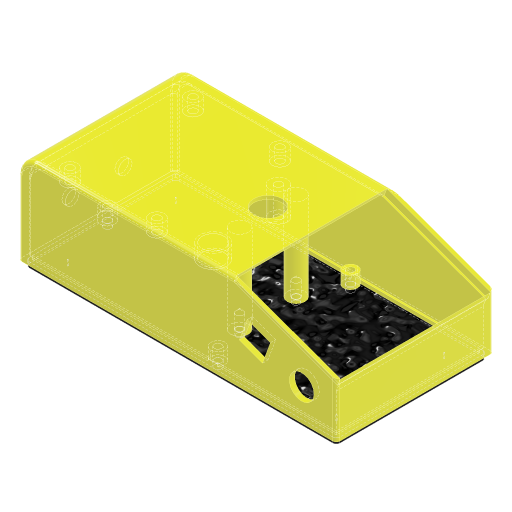
# Autodesk Inventor part: gabinete6
Saved by Autodesk Inventor 2023 (Build 270158000, 158)
## iProperties
Created: 2023-09-18
Part Number: gabinete6
Material: Generic
Document SubType Name: Modeling
Designer: Claudimir
Density: 1 g/cm^3
Appearance: Default
Author: Claudimir
Autodesk Inventor part; units mm, degrees
ref_plane "YZ Plane" through (0, 0, 0) normal (1, 0, 0) x (0, 1, 0)
ref_plane "XZ Plane" through (0, 0, 0) normal (0, 1, 0) x (-1, 0, 0)
sketch "Sketch1" plane through (0, 0, 0) normal (0, 0, 1) x (1, 0, 0)
  line L0 (0, 0) -> (9.2345, 25.3717) construction
  line L1 (9.2345, 25.3717) -> (-49.0264, 46.5769)
  line L2 (-49.0264, 46.5769) -> (-58.2609, 21.2052) construction
  line L3 (-58.2609, 21.2052) -> (0, 0) construction
  line L4 (-49.0264, 46.5769) -> (-53.6437, 33.8911) construction
  line L5 (-53.6437, 33.8911) -> (-40.9578, 29.2738) construction
  line L6 (-40.9578, 29.2738) -> (-36.3405, 41.9597) construction
  line L7 (-36.3405, 41.9597) -> (-49.0264, 46.5769) construction
  line L8 (-40.9578, 29.2738) -> (-45.0621, 17.9975) construction
  line L9 (-45.0621, 17.9975) -> (-32.8461, 13.5513) construction
  line L10 (-32.8461, 13.5513) -> (-28.7418, 24.8276) construction
  line L11 (-28.7418, 24.8276) -> (-40.9578, 29.2738) construction
  line L12 (9.2345, 25.3717) -> (4.4463, 12.216) construction
  line L13 (4.4463, 12.216) -> (-4.011, 15.2942) construction
  line L14 (-4.011, 15.2942) -> (0.7773, 28.4499) construction
  line L15 (0.7773, 28.4499) -> (9.2345, 25.3717) construction
  line L16 (-4.011, 15.2942) -> (-7.4312, 5.8973) construction
  line L17 (-7.4312, 5.8973) -> (-16.8281, 9.3175) construction
  line L18 (-16.8281, 9.3175) -> (-13.4079, 18.7144) construction
  line L19 (-13.4079, 18.7144) -> (-4.011, 15.2942) construction
  line L20 (-170.7655, -8.4231) -> (9.2345, -8.4231)
  line L21 (9.2345, -8.4231) -> (9.2345, 25.3717)
  line L22 (-49.0264, 46.5769) -> (-170.7655, 46.5769)
  line L23 (-45.7029, 17.6987) -> (-41.2567, 29.9147)
  line L24 (-41.2567, 29.9147) -> (-28.101, 25.1264)
  line L25 (-28.101, 25.1264) -> (-32.5472, 12.9104)
  line L26 (-32.5472, 12.9104) -> (-45.7029, 17.6987)
  line L27 (-13.4079, 18.7144) -> (-7.4312, 5.8973) construction
  line L28 (-4.011, 15.2942) -> (-16.8281, 9.3175) construction
  circle A0 centre (-10.4195, 12.3058) radius 7
  line L29 (-170.7655, 46.5769) -> (-170.7655, -8.4231)
  line L30 (-168.7655, 44.5769) -> (-49.7543, 44.5769)
  line L31 (6.2345, 17.1293) -> (6.2345, -8.4231)
  line L32 (-168.7655, -8.4231) -> (-168.7655, 44.5769)
  line L33 (-49.7543, 44.5769) -> (-49.0264, 46.5769)
  line L34 (6.2345, 17.1293) -> (9.2345, 25.3717)
  point P0 (6.2345, -8.4231)
  dimension "d0" = 27
  dimension "d1" = 62
  dimension "d4" = 12
  dimension "d5" = 13
  dimension "d6" = 14
  dimension "d7" = 9
  dimension "d8" = 10
  dimension "d9" = 10
  dimension "d13" = 180
  dimension "d17" = 0.5
  dimension "d18" = 14
  dimension "d19" = 55
  dimension "d22" = 2
  constraints: 70 end point, 13 parallel, 6 perpendicular, 3 point on line, 1 centre point, 1 collinear, 1 horizontal, 1 midpoint, 1 vertical, 5 other
  measures "d0" distance of L2.end L1.end
  measures "d1" distance of L1.end L0.end
  measures "d4" distance of L10.end L9.end
  measures "d5" distance of L9.end L8.end
  measures "d6" distance of L13.end L14.end
  measures "d7" distance of L12.end L13.end
  measures "d8" distance of L17.end L18.end
  measures "d9" distance of L16.end L17.end
  measures "d13" distance of L20.end L20.start
  measures "d17" distance between parallel lines of L8 L23
  measures "d18" diameter of A0
  measures "d19" distance of L22.end L20.start
  measures "d22" distance between parallel lines of L22 L30
extrude "corpo 1" add sketch "Sketch1" against normal blind 89 contours L34 L31 L20 L32 L30 L33 L1 | L21 L20 L31 L34 | L33 L30 L32 L20 L29 L22 | L23 L24 L25 L26 | A0
extrude "corpo 2" cut sketch "Sketch1" against normal blind 86 contours L34 L31 L20 L32 L30 L33 L1 | L23 L24 L25 L26 | A0
extrude "corpo 3" add sketch "Sketch1" against normal blind 3
sketch "Sketch2" plane through (-170.7655, 46.5769, -89) normal (0, 1, 0) x (1, 0, 0)
  line L0 (121.7391, 0) -> (180, 0) construction
  line L1 (121.7391, 0) -> (96.7391, 0) construction
  line L2 (96.7391, 0) -> (96.7391, -44.5) construction
  line L3 (96.7391, -44.5) -> (121.7391, -44.5) construction
  line L4 (121.7391, -44.5) -> (121.7391, 0) construction
  circle A0 centre (96.7391, -44.5) radius 8
  point P0 (170.7655, -89)
  dimension "d27" = 25
  dimension "d28" = 44.5
  dimension "d29" = 16
  constraints: 8 end point, 2 parallel, 1 centre point, 1 coincident, 1 horizontal, 1 perpendicular
  measures "d27" distance of L3.end L2.end
  measures "d28" distance of L2.end L1.end
  measures "d29" diameter of A0
extrude "Extrusion6" cut sketch "Sketch2" against normal through all
sketch "Sketch3" plane through (-170.7655, -8.4231, 0) normal (-1, 0, 0) x (0, 0, 1)
  line L0 (0, 0) -> (-87, 0) construction
  line L1 (-87, 0) -> (-87, 20) construction
  line L2 (-87, 20) -> (0, 20) construction
  line L3 (0, 20) -> (0, 0) construction
  line L4 (-58.5, 16) -> (-28.5, 16) construction
  line L5 (-28.5, 16) -> (-28.5, 24) construction
  line L6 (-28.5, 24) -> (-58.5, 24) construction
  line L7 (-58.5, 24) -> (-58.5, 16) construction
  line L8 (-58.5, 16) -> (-28.5, 24) construction
  line L9 (-28.5, 16) -> (-58.5, 24) construction
  circle A0 centre (-58.5, 20) radius 3.9
  circle A1 centre (-28.5, 20) radius 3.9
  point P0 (-43.5, 20)
  dimension "d32" = 20
  dimension "d33" = 30
  dimension "d35" = 7.8
  dimension "d36" = 7.8
  constraints: 20 end point, 5 midpoint, 4 parallel, 2 centre point, 2 horizontal, 2 perpendicular
  measures "d32" distance of L0.end L1.end
  measures "d33" distance of L6.end L5.end
  measures "d35" diameter of A0
  measures "d36" diameter of A1
extrude "Extrusion7" cut sketch "Sketch3" against normal up to surface (2 mm away)
sketch "Sketch4" plane through (-168.7655, 44.5769, -86) normal (0, -1, 0) x (1, 0, 0)
  circle A0 centre (94.7391, 41.5) radius 8 construction
  line L0 (86.7391, 41.5) -> (66.7391, 41.5) construction
  line L1 (66.7391, 41.5) -> (66.7391, 76.3) construction
  line L2 (66.7391, 76.3) -> (86.7391, 76.3) construction
  line L3 (86.7391, 76.3) -> (86.7391, 41.5) construction
  line L4 (66.7391, 76.3) -> (17.5391, 76.3) construction
  line L5 (17.5391, 76.3) -> (17.5391, 6.7) construction
  line L6 (17.5391, 6.7) -> (66.7391, 6.7) construction
  line L7 (66.7391, 6.7) -> (66.7391, 76.3) construction
  line L8 (94.7391, 41.5) -> (94.7391, 57.5) construction
  circle A1 centre (94.7391, 41.5) radius 11 construction
  line L9 (94.7391, 41.5) -> (94.7391, 25.5) construction
  circle A2 centre (94.7391, 57.5) radius 5
  circle A3 centre (94.7391, 25.5) radius 5
  circle A4 centre (17.5391, 76.3) radius 4.25
  circle A5 centre (17.5391, 6.7) radius 4.25
  circle A6 centre (66.7391, 76.3) radius 4.25
  circle A7 centre (66.7391, 6.7) radius 4.25
  circle A8 centre (94.7391, 57.5) radius 2.15
  circle A9 centre (94.7391, 25.5) radius 2.15
  line L10 (94.7391, 57.5) -> (94.7391, 72.5) construction
  circle A10 centre (94.7391, 72.5) radius 6.2
  circle A11 centre (94.7391, 72.5) radius 7.5
  line L11 (94.7391, 25.5) -> (84.7391, 25.5) construction
  circle A12 centre (84.7391, 25.5) radius 5
  circle A13 centre (84.7391, 25.5) radius 2.15
  point P0 (168.7655, 86)
  point P1 (14.075, 76.3)
  point P2 (70.2032, 76.3)
  point P3 (14.075, 6.7)
  dimension "d40" = 20
  dimension "d41" = 34.8
  dimension "d42" = 49.2
  dimension "d43" = 69.6
  dimension "d44" = 16
  dimension "d45" = 22
  dimension "d46" = 16
  dimension "d47" = 10
  dimension "d48" = 10
  dimension "d51" = 8.5
  dimension "d52" = 8.5
  dimension "d53" = 8.5
  dimension "d54" = 8.5
  dimension "d59" = 4.3
  dimension "d60" = 4.3
  dimension "d82" = 15
  dimension "d83" = 12.4
  dimension "d84" = 15
  dimension "d131" = 10
  dimension "d132" = 4.3
  constraints: 24 end point, 19 coincident, 13 centre point, 4 parallel, 3 perpendicular, 3 point on line, 3 vertical, 2 horizontal, 1 equal radius, 1 horizontal alignment, 1 other
  measures "d40" distance of L1.end L2.end
  measures "d41" distance of L0.end L1.end
  measures "d42" distance of L6.end L5.end
  measures "d43" distance of L5.end L4.end
  measures "d44" distance of L8.start L8.end
  measures "d45" diameter of A1
  measures "d46" distance of L9.start L9.end
  measures "d47" diameter of A2
  measures "d48" diameter of A3
  measures "d51" diameter of A4
  measures "d52" diameter of A5
  measures "d53" diameter of A6
  measures "d54" diameter of A7
  measures "d59" diameter of A8
  measures "d60" diameter of A9
  measures "d82" distance of L10.start L10.end
  measures "d83" diameter of A10
  measures "d84" diameter of A11
  measures "d131" distance of L11.start L11.end
  measures "d132" diameter of A13
extrude "pilares" add sketch "Sketch4" along normal blind 50 contours A2 | A3 | A8 | A9
sketch "Sketch8" plane through (-74.0264, -5.4231, -28.5) normal (0, -1, 0) x (1, 0, 0)
  circle A0 centre (0, 0) radius 5 projected
  circle A1 centre (0, 0) radius 2.15
  circle A2 centre (0, -32) radius 5 projected
  circle A3 centre (0, -32) radius 2.15
  point P0 (74.0264, 28.5)
  dimension "d104" = 4.3
  dimension "d105" = 4.3
  constraints: 2 centre point, 2 coincident
  measures "d104" diameter of A1
  measures "d105" diameter of A3
extrude "parafuso pilar" cut sketch "Sketch8" against normal blind 10 contours A1 | A3
chamfer "Chamfer1" distance 2 angle 45 2 edges at (-76.1764, 4.5769, -28.5) (-76.1764, 4.5769, -60.5)
extrude "Extrusion12" add sketch "Sketch4" along normal blind 7 contours A4 | A5 | A6 | A7
sketch "Sketch9" plane through (-151.2264, 37.5769, -79.3) normal (0, -1, 0) x (1, 0, 0)
  circle A0 centre (49.2, 69.6) radius 4.25 projected
  circle A1 centre (49.2, 69.6) radius 2.15
  circle A2 centre (0, 69.6) radius 4.25 projected
  circle A3 centre (0, 69.6) radius 2.15
  circle A4 centre (0, 0) radius 4.25 projected
  circle A5 centre (0, 0) radius 2.15
  circle A6 centre (49.2, 0) radius 4.25 projected
  circle A7 centre (49.2, 0) radius 2.15
  point P0 (151.2264, 79.3)
  dimension "d111" = 4.3
  dimension "d112" = 4.3
  dimension "d113" = 4.3
  dimension "d114" = 4.3
  constraints: 4 centre point, 4 coincident
  measures "d111" diameter of A1
  measures "d112" diameter of A3
  measures "d113" diameter of A5
  measures "d114" diameter of A7
extrude "Extrusion22" cut sketch "Sketch9" against normal blind 7 contours A1 | A3 | A5 | A7
extrude "Extrusion15" add sketch "Sketch4" along normal blind 8 contours A11
fillet "Fillet1" radius 10 2 edges at (-168.7655, 44.5769, -44.5) (-170.7655, 46.5769, -44.5)
sketch "Sketch5" plane through (-170.7655, -8.4231, 0) normal (0, -1, 0) x (1, 0, 0)
  line L0 (0, 0) -> (0, -89) projected
  line L1 (121.7391, -89) -> (180, -89) projected
  line L2 (0, 0) -> (180, 0)
  line L3 (180, 0) -> (180, -89)
  line L4 (180, -89) -> (0, -89)
  line L5 (0, -89) -> (0, 0)
  line L6 (176, -4) -> (4, -4)
  line L7 (4, -4) -> (4, -85)
  line L8 (4, -85) -> (176, -85)
  line L9 (176, -85) -> (176, -4)
  line L10 (177, -3) -> (3, -3)
  line L11 (3, -3) -> (3, -86)
  line L12 (3, -86) -> (177, -86)
  line L13 (177, -86) -> (177, -3)
  point P0 (170.7655, 0)
  point P1 (0, -86)
  dimension "d87" = 4
  dimension "d88" = 3
  constraints: 24 end point, 6 parallel, 3 perpendicular, 1 horizontal, 6 other
  measures "d87" distance between parallel lines of L2 L6
  measures "d88" distance between parallel lines of L2 L10
extrude "Extrusion16" add sketch "Sketch5" against normal blind 5 contours L2 L3 L1 L4 L0 | L13 L12 L11 L10
extrude "Extrusion17" cut sketch "Sketch5" against normal up to surface (3 mm away) contours L13 L12 L11 L10
sketch "Sketch6" plane through (-170.7655, -8.4231, 0) normal (0, -1, 0) x (1, 0, 0)
  line L0 (4, -4) -> (4, -85) construction
  line L1 (4, -44.5) -> (6, -44.5) construction
  circle A0 centre (6, -44.5) radius 2.1
  circle A1 centre (6, -44.5) radius 4
  line L2 (6, -44.5) -> (106, -44.5) construction
  line L3 (106, -44.5) -> (106, -7) construction
  line L4 (106, -7) -> (6, -7) construction
  line L5 (6, -7) -> (6, -44.5) construction
  line L6 (6, -44.5) -> (106, -44.5) construction
  line L7 (106, -44.5) -> (106, -82) construction
  line L8 (106, -82) -> (6, -82) construction
  line L9 (6, -82) -> (6, -44.5) construction
  circle A2 centre (106, -7) radius 2.1
  circle A3 centre (106, -7) radius 4
  circle A4 centre (106, -82) radius 2.1
  circle A5 centre (106, -82) radius 4
  point P0 (170.7655, 0)
  dimension "d93" = 2
  dimension "d94" = 4.2
  dimension "d95" = 8
  dimension "d135" = 100
  dimension "d136" = 37.5
  dimension "d138" = 37.5
  dimension "d139" = 4.2
  dimension "d140" = 8
  dimension "d141" = 4.2
  dimension "d142" = 8
  constraints: 18 end point, 6 centre point, 6 coincident, 4 parallel, 3 horizontal, 2 perpendicular, 1 midpoint
  measures "d93" distance of L1.start L1.end
  measures "d94" diameter of A0
  measures "d95" diameter of A1
  measures "d135" distance of L4.end L3.end
  measures "d136" distance of L3.end L2.end
  measures "d138" distance of L6.end L7.end
  measures "d139" diameter of A2
  measures "d140" diameter of A3
  measures "d141" diameter of A4
  measures "d142" diameter of A5
extrude "parafuso lateral" add sketch "Sketch6" against normal blind 10 contours A0 | A1 | A2 | A3 | A4 | A5
extrude "parafuso lateral 2" cut sketch "Sketch6" against normal blind 10 contours A0 | A2 | A4
ref_plane "Work Plane1" through (-49.0264, 46.5769, -86) normal (0.3420201, 0.9396926, 0) x (0, 0, 1)
sketch "Sketch7" plane through (-49.0264, 46.5769, -86) normal (0.3420201, 0.9396926, 0) x (0, 0, 1)
  line L0 (83, 0) -> (0, 0) construction
  line L1 (0, 70.7394) -> (0, -92.7671) construction
  line L2 (83, 0) -> (0, 0) construction
  line L3 (0, 0) -> (0, 62) construction
  line L4 (0, 62) -> (83, 62) construction
  line L5 (83, 62) -> (83, 0) construction
  line L6 (83, 0) -> (0, 62) construction
  line L7 (83, 62) -> (0, 62) construction
  line L8 (83, 62) -> (0, 0) construction
  line L9 (84, 62.2) -> (-1, 62.2)
  line L10 (-1, 62.2) -> (-1, -0.2)
  line L11 (-1, -0.2) -> (84, -0.2)
  line L12 (84, -0.2) -> (84, 62.2)
  line L13 (84, 62.2) -> (-1, -0.2) construction
  line L14 (-1, 62.2) -> (84, -0.2) construction
  point P0 (86, 62)
  point P1 (41.5, 31)
  point P2 (0, -93.7068)
  dimension "d100" = 85
  dimension "d101" = 62.4
  constraints: 24 end point, 4 parallel, 3 midpoint, 2 horizontal, 2 perpendicular, 1 point on line
  measures "d100" distance of L11.end L10.end
  measures "d101" distance of L10.end L9.end
extrude "janela" cut sketch "Sketch7" against normal blind 4.2
fillet "Fillet3" radius 2 6 edges at (-167.8365, 43.648, 0) (-170.7655, 14.0769, 0) (-104.8959, 46.5769, 0) (-167.8365, 43.648, -89) (-170.7655, 14.0769, -89) (-104.8959, 46.5769, -89)
fillet "Fillet4" radius 2 6 edges at (-165.8365, 41.648, -86) (-168.7655, 15.5769, -86) (-104.3663, 44.5769, -86) (-165.8365, 41.648, -3) (-168.7655, 15.5769, -3) (-104.3663, 44.5769, -3)
sketch "Sketch10" plane through (9.2345, -8.4231, -89) normal (0, -1, 0) x (1, 0, 0)
  line L0 (0, 0) -> (-181, 0)
  line L1 (-181, 0) -> (-181, 90)
  line L2 (-181, 90) -> (0, 90)
  line L3 (0, 90) -> (0, 0)
  point P0 (-9.2345, 89)
  dimension "d119" = 181
  dimension "d120" = 90
  constraints: 8 end point, 2 parallel, 1 horizontal, 1 perpendicular
  measures "d119" distance of L1.end L2.end
  measures "d120" distance of L0.end L1.end
extrude "Extrusion23" cut sketch "Sketch10" against normal up to surface (3 mm away)
fillet "Fillet5" radius 2 2 edges at (9.2345, 9.9743, 0) (9.2345, 9.9743, -89)
extrude "Extrusion25" add sketch "Sketch4" along normal blind 16 contours A12
sketch "Sketch11" plane through (-170.7655, -5.4231, -87) normal (0, -1, 0) x (1, 0, 0)
  line L0 (4, 83) -> (4, 45.9641) construction
  line L1 (4, 2) -> (176, 2) construction
  line L2 (4, 83) -> (176, 83) construction
  line L3 (176, 83) -> (176, 2) construction
  line L4 (176, 2) -> (4, 2) construction
  line L5 (4, 2) -> (4, 83) construction
  line L6 (176, 85) -> (4, 85)
  line L7 (2, 83) -> (2, 2)
  line L8 (4, 0) -> (176, 0)
  line L9 (178, 2) -> (178, 83)
  circle A0 centre (6, 42.5) radius 2.1 projected
  circle A1 centre (6, 42.5) radius 1.9
  circle A2 centre (96.7391, 58.5) radius 1.9
  circle A3 centre (96.7391, 26.5) radius 1.9
  arc A4 (4, 85) -> (2, 83) centre (4, 83) ccw
  arc A5 (178, 83) -> (176, 85) centre (176, 83) ccw
  arc A6 (176, 0) -> (178, 2) centre (176, 2) ccw
  arc A7 (2, 2) -> (4, 0) centre (4, 2) ccw
  circle A8 centre (106, 80) radius 2.1 projected
  circle A9 centre (106, 5) radius 2.1 projected
  line L10 (14, 12) -> (2, 12) construction
  line L11 (2, 12) -> (2, 0) construction
  line L12 (2, 0) -> (14, 0) construction
  line L13 (14, 0) -> (14, 12) construction
  line L14 (2, 85) -> (14, 85) construction
  line L15 (14, 85) -> (14, 73) construction
  line L16 (14, 73) -> (2, 73) construction
  line L17 (2, 73) -> (2, 85) construction
  line L18 (178, 85) -> (166, 85) construction
  line L19 (166, 85) -> (166, 73) construction
  line L20 (166, 73) -> (178, 73) construction
  line L21 (178, 73) -> (178, 85) construction
  line L22 (178, 0) -> (166, 0) construction
  line L23 (166, 0) -> (166, 12) construction
  line L24 (166, 12) -> (178, 12) construction
  line L25 (178, 12) -> (178, 0) construction
  circle A10 centre (14, 73) radius 0.25
  circle A11 centre (14, 12) radius 0.25
  circle A12 centre (166, 73) radius 0.25
  circle A13 centre (166, 12) radius 0.25
  point P0 (170.7655, 87)
  dimension "d124" = 2
  dimension "d125" = 3.8
  dimension "d126" = 3.8
  dimension "d127" = 3.8
  dimension "d130" = 2
  dimension "d145" = 12
  dimension "d146" = 12
  dimension "d147" = 12
  dimension "d148" = 12
  dimension "d149" = 12
  dimension "d150" = 12
  dimension "d151" = 0.5
  dimension "d152" = 0.5
  dimension "d153" = 0.5
  dimension "d154" = 0.5
  constraints: 48 end point, 12 parallel, 11 centre point, 8 point on circle, 8 point on line, 8 tangent, 7 coincident, 6 perpendicular, 5 horizontal, 3 equal radius, 3 other
  measures "d124" distance between parallel lines of L2 L6
  measures "d125" diameter of A1
  measures "d126" diameter of A2
  measures "d127" diameter of A3
  measures "d130" radius of A4
  measures "d145" distance of L15.end L16.end
  measures "d146" distance of L14.end L15.end
  measures "d147" distance of L20.end L19.end
  measures "d148" distance of L19.end L18.end
  measures "d149" distance of L23.end L24.end
  measures "d150" distance of L22.end L23.end
  measures "d151" diameter of A10
  measures "d152" diameter of A11
  measures "d153" diameter of A12
  measures "d154" diameter of A13
extrude "Extrusion27" add sketch "Sketch11" along normal blind 3 separate body contours A5 L9 A6 L8 A7 L7 A4 L6
equation "\"d28\" = 0.5 * d20"
equation "\"d36\" = d35"
equation "\"d52\" = d51"
equation "\"d53\" = d51"
equation "\"d54\" = d51"
equation "\"d112\" = d111"
equation "\"d113\" = d111"
equation "\"d114\" = d111"
equation "\"d20\" = 89"
